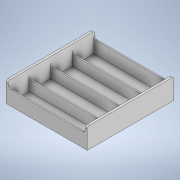
# Autodesk Inventor part: BatteryCompartment
Saved by Autodesk Inventor 2021 (Build 250183000, 183)
## iProperties
Created: 2022-01-13
Part Number: BatteryCompartment
Material: Типовые
Document SubType Name: Modeling
Designer: Maxim
Density: 1 g/cm^3
Appearance: По умолчанию
Author: Maxim
Autodesk Inventor part; units mm, degrees
ref_plane "YZ Plane" through (0, 0, 0) normal (1, 0, 0) x (0, 1, 0)
ref_plane "XZ Plane" through (0, 0, 0) normal (0, 1, 0) x (-1, 0, 0)
ref_plane "XY Plane" through (0, 0, 0) normal (0, 0, 1) x (1, 0, 0)
sketch "Эскиз1" plane through (0, 0, 0) normal (0, 1, 0) x (-1, 0, 0)
  line L0 (0, 0) -> (-75, 0)
  line L1 (-75, 0) -> (-75, 80)
  line L2 (-75, 80) -> (0, 80)
  line L3 (0, 80) -> (0, 0)
  line L4 (0, 60) -> (-75, 60)
  line L5 (0, 61) -> (-75, 61)
  line L6 (0, 79) -> (-75, 79)
  line L7 (0, 40) -> (-75, 40)
  line L8 (-75, 20) -> (0, 20)
  line L9 (0, 1) -> (-75, 1)
  line L10 (0, 21) -> (-75, 21)
  line L11 (0, 41) -> (-75, 41)
  line L12 (-2, 80) -> (-2, 0)
  line L13 (-73, 0) -> (-73, 80)
  point P0 (-73, 20)
  point P1 (-73, 1)
  point P2 (-2, 1)
  point P3 (-2, 20)
  point P4 (-73, 40)
  point P5 (-73, 21)
  point P6 (-2, 21)
  point P7 (-2, 40)
  point P8 (-73, 60)
  point P9 (-73, 41)
  point P10 (-2, 41)
  point P11 (-2, 60)
  point P12 (-73, 79)
  point P13 (-73, 61)
  point P14 (-2, 61)
  point P15 (-2, 79)
  dimension "d0" = 75
  dimension "d1" = 80
  dimension "d2" = 20
  dimension "d3" = 1
  dimension "d4" = 1
  dimension "d5" = 20
  dimension "d6" = 20
  dimension "d7" = 19
  dimension "d8" = 1
  dimension "d9" = 1
  dimension "d10" = 2
  dimension "d11" = 2
  constraints: 24 end point, 10 horizontal, 4 point on line, 2 perpendicular, 1 parallel, 22 other
  measures "d0" distance of L2.start L2.end
  measures "d1" distance of L0.end L2.start
  measures "d2" distance between parallel lines of L2 L4
  measures "d3" distance between parallel lines of L4 L5
  measures "d4" distance between parallel lines of L2 L6
  measures "d5" distance between parallel lines of L7 L4
  measures "d6" distance between parallel lines of L7 L8
  measures "d7" distance between parallel lines of L8 L9
  measures "d8" distance between parallel lines of L7 L11
  measures "d9" distance between parallel lines of L8 L10
  measures "d10" distance of the line from the sketch origin of L12
extrude "Выдавливание1" add sketch "Эскиз1" along normal blind 1 contours L9 L13 L8 L12 | L10 L13 L7 L12 | L11 L13 L4 L12 | L5 L13 L6 L12
extrude "Выдавливание2" add sketch "Эскиз1" along normal blind 19 contours L0 L12 L9 L3 | L9 L12 L8 L3 | L0 L1 L9 L13 | L8 L12 L10 L3 | L9 L1 L8 L13 | L10 L12 L7 L3 | L8 L1 L10 L13 | L7 L12 L11 L3 | L10 L1 L7 L13 | L11 L12 L4 L3 | L7 L1 L11 L13 | L4 L12 L5 L3 | L11 L1 L4 L13 | L5 L12 L6 L3 | L4 L1 L5 L13 | L6 L12 L2 L3 | L5 L1 L6 L13 | L6 L1 L2 L13
extrude "Выдавливание3" add sketch "Эскиз1" along normal blind 13 contours L0 L13 L9 L12 | L6 L13 L2 L12
extrude "Выдавливание4" add sketch "Эскиз1" along normal blind 11 contours L8 L13 L10 L12 | L7 L13 L11 L12 | L4 L13 L5 L12
fillet "Сопряжение1" radius 2 4 edges at (1, 19, 80) (1, 19, 0) (74, 19, 0) (74, 19, 80)
fillet "Сопряжение2" radius 2 10 edges at (2, 13, 79.5) (2, 11, 20.5) (2, 11, 40.5) (2, 11, 60.5) (2, 13, 0.5) (73, 13, 0.5) (73, 11, 20.5) (73, 11, 40.5) (73, 11, 60.5) (73, 13, 79.5)
